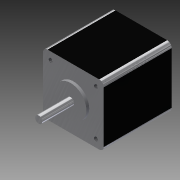
# Autodesk Inventor part: CNC- Stepper Motor
Saved by Autodesk Inventor 2015 (Build 190159000, 159)
## iProperties
Created: 2015-03-20
Part Number: CNC- Stepper Motor
Material: Generic
Document SubType Name: Modeling
Designer: Bangladesh
Density: 1 g/cm^3
Appearance: Default
Author: Bangladesh
Autodesk Inventor part; units mm, degrees
ref_plane "YZ Plane" through (0, 0, 0) normal (1, 0, 0) x (0, 1, 0)
ref_plane "XZ Plane" through (0, 0, 0) normal (0, 1, 0) x (-1, 0, 0)
ref_plane "XY Plane" through (0, 0, 0) normal (0, 0, 1) x (1, 0, 0)
sketch "Sketch1" plane through (0, 0, 0) normal (0, 0, 1) x (1, 0, 0)
  line L0 (-21.125, 21.125) -> (21.125, 21.125)
  line L1 (21.125, 21.125) -> (21.125, -21.125)
  line L2 (21.125, -21.125) -> (-21.125, -21.125)
  line L3 (-21.125, -21.125) -> (-21.125, 21.125)
  line L4 (-21.125, 21.125) -> (21.125, -21.125) construction
  line L5 (21.125, 21.125) -> (-21.125, -21.125) construction
  point P0 (0, 0)
  dimension "d0" = 42.25
  dimension "d1" = 42.25
  constraints: 12 end point, 2 midpoint, 2 parallel, 1 horizontal, 1 perpendicular
  measures "d0" distance of L0.end L1.end
  measures "d1" distance of L1.end L2.end
extrude "Extrusion1" add sketch "Sketch1" along normal mid plane 47.18
sketch "Sketch2" plane through (0, 0, 23.59) normal (0, 0, 1) x (1, 0, 0)
  circle A0 centre (0, 0) radius 11
  dimension "d4" = 22
  constraints: 1 centre point, 1 coincident
  measures "d4" diameter of A0
extrude "Extrusion2" add sketch "Sketch2" along normal blind 1.97
fillet "Fillet1" radius 3.175 4 edges at (-21.125, 21.125, 0) (-21.125, -21.125, 0) (21.125, 21.125, 0) (21.125, -21.125, 0)
sketch "Sketch3" plane through (0, 0, 25.56) normal (0, 0, 1) x (1, 0, 0)
  circle A0 centre (0, 0) radius 2.5
  dimension "d8" = 5
  constraints: 1 centre point, 1 coincident
  measures "d8" diameter of A0
extrude "Extrusion3" add sketch "Sketch3" along normal blind 22.15
sketch "Sketch4" plane through (0, 0, -23.59) normal (0, 0, -1) x (-1, 0, 0)
  circle A0 centre (-15.76, 15.76) radius 2.95
  circle A1 centre (15.76, 15.76) radius 2.95
  circle A2 centre (-15.76, -15.76) radius 2.95
  circle A3 centre (15.76, -15.76) radius 2.95
  line L0 (-21.125, 17.95) -> (-21.125, -17.95) projected
  line L1 (17.95, 21.125) -> (-17.95, 21.125) projected
  line L2 (21.125, -17.95) -> (21.125, 17.95) projected
  line L3 (-17.95, -21.125) -> (17.95, -21.125) projected
  point P0 (0, 0)
  dimension "d12" = 5.9
  dimension "d13" = 5.9
  dimension "d14" = 5.9
  dimension "d16" = 5.365
  dimension "d17" = 5.365
  dimension "d18" = 5.365
  dimension "d19" = 5.365
  constraints: 4 centre point
  measures "d12" diameter of A1
  measures "d13" diameter of A2
  measures "d14" diameter of A3
  measures "d16" distance from line of L0 A0.centre
  measures "d17" distance from line of L1 A0.centre
  measures "d18" distance from line of L2 A3.centre
  measures "d19" distance from line of L3 A3.centre
hole "Hole1" at (15.76, 15.76, -23.59) at (-15.76, 15.76, -23.59) at (-15.76, -15.76, -23.59) at (15.76, -15.76, -23.59) direction (0, 0, 1) diameter 5.9 depth 2.2
sketch "Sketch7" plane through (15.76, -15.76, -21.39) normal (0, 0, -1) x (-1, 0, 0)
  circle A0 centre (0, 0) radius 1.524
  point P0 (15.76, 15.76)
  dimension "d46" = 3.048
  constraints: 1 centre point
  measures "d46" diameter of A0
hole "Hole3" at (15.76, -15.76, -21.39) direction (0, 0, 1) diameter 2.8194 end through all thread size "6-40 UNF" class "2B" standard "ANSI Unified Screw Threads"
sketch "Sketch8" plane through (15.76, 15.76, -21.39) normal (0, 0, -1) x (-1, 0, 0)
  circle A0 centre (0, 0) radius 1.524
  point P0 (15.76, -15.76)
  dimension "d54" = 3.048
  constraints: 1 centre point
  measures "d54" diameter of A0
hole "Hole4" at (15.76, 15.76, -21.39) direction (0, 0, 1) diameter 2.8194 end through all thread size "6-40 UNF" class "2B" standard "ANSI Unified Screw Threads"
sketch "Sketch9" plane through (-15.76, -15.76, -21.39) normal (0, 0, -1) x (-1, 0, 0)
  circle A0 centre (0, 0) radius 1.524
  point P0 (-15.76, 15.76)
  dimension "d62" = 3.048
  constraints: 1 centre point
  measures "d62" diameter of A0
hole "Hole5" at (-15.76, -15.76, -21.39) direction (0, 0, 1) diameter 2.8194 end through all thread size "6-40 UNF" class "2B" standard "ANSI Unified Screw Threads"
sketch "Sketch10" plane through (-15.76, 15.76, -21.39) normal (0, 0, -1) x (-1, 0, 0)
  circle A0 centre (0, 0) radius 1.524
  point P0 (-15.76, -15.76)
  dimension "d70" = 3.048
  constraints: 1 centre point
  measures "d70" diameter of A0
hole "Hole6" at (-15.76, 15.76, -21.39) direction (0, 0, 1) diameter 2.8194 end through all thread size "6-40 UNF" class "2B" standard "ANSI Unified Screw Threads"
equation "\"d1\" = d0"
body "Solid1"
